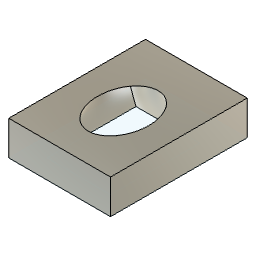
toothbrush_charger_case (Autodesk Fusion 360 design; units mm, degrees)
Autodesk Fusion 360 part; units mm, degrees
sketch "Sketch1" plane through (0, 0, 0) normal (0, 0, 1) x (1, 0, 0)
  line L0 (0, 0) -> (-70, 0)
  line L1 (-70, 0) -> (-70, 90)
  line L2 (-70, 90) -> (0, 90)
  line L3 (0, 90) -> (0, 0)
  line L4 (-70, 0) -> (0, 0)
  line L5 (0, 0) -> (0, 10)
  line L6 (0, 10) -> (-70, 10)
  line L7 (-70, 10) -> (-70, 0)
  line L8 (-70, 10) -> (-35, 10)
  line L9 (0, 10) -> (0, 32.5)
  line L10 (-35, 10) -> (-15, 10)
  line L11 (-15, 10) -> (-15, 37.5)
  line L12 (-15, 10) -> (-35, 10)
  line L13 (-35, 10) -> (-35, 37.5)
  line L14 (-35, 37.5) -> (-15, 37.5)
  line L15 (-15, 37.5) -> (-15, 10)
  ellipse E0 centre (-35, 37.5) end of major axis (-35, 10) minor radius 20
  line L16 (-35, 65) -> (-35, 10) construction
  line L17 (-55, 37.5) -> (-15, 37.5) construction
  line L18 (0, 10) -> (-10, 10)
  line L19 (-10, 10) -> (-60, 10)
  line L20 (-60, 10) -> (-60, 72.5)
  line L21 (-60, 72.5) -> (-10, 72.5)
  line L22 (-10, 72.5) -> (-10, 10)
  line L23 (0, 10) -> (-70, 10)
  line L24 (-70, 10) -> (-70, 2.5)
  line L25 (-70, 2.5) -> (0, 2.5)
  line L26 (0, 2.5) -> (0, 10)
  line L27 (0, 2.5) -> (-70, 2.5)
  line L28 (-70, 2.5) -> (-70, -7.5)
  line L29 (-70, -7.5) -> (0, -7.5)
  line L30 (0, -7.5) -> (0, 2.5)
  line L31 (-10, 10) -> (-60, 10)
  line L32 (-60, 10) -> (-60, 2.5)
  line L33 (-60, 2.5) -> (-10, 2.5)
  line L34 (-10, 2.5) -> (-10, 10)
  line L35 (0, -7.5) -> (5, -7.5)
  line L36 (5, -7.5) -> (5, -12.5)
  line L37 (5, -12.5) -> (0, -12.5)
  line L38 (0, -12.5) -> (0, -7.5)
  line L39 (5, -12.5) -> (-75, -12.5)
  line L40 (-75, -12.5) -> (-75, 95)
  line L41 (-75, 95) -> (5, 95)
  line L42 (5, 95) -> (5, -12.5)
  dimension "d1" = 70
  dimension "d2" = 90
  dimension "d3" = 10
  dimension "d4" = 35
  dimension "d5" = 22.5
  dimension "d6" = 20
  dimension "d7" = 27.5
  dimension "d8" = 27.5
  dimension "d11" = 10
  dimension "d12" = 50
  dimension "d13" = 62.5
  dimension "d14" = 70
  dimension "d15" = 7.5
  dimension "d16" = 70
  dimension "d17" = 10
  dimension "d20" = 50
  dimension "d21" = 7.5
  dimension "d22" = 5
  dimension "d23" = 5
  dimension "d24" = 80
  dimension "d25" = 107.5
  constraint horizontal L0
  constraint vertical L1
  constraint horizontal L2
  constraint vertical L3
  constraint coincident L0.start L3.end
  constraint horizontal L4
  constraint vertical L5
  constraint horizontal L6
  constraint vertical L7
  constraint perpendicular L7 L8
  constraint perpendicular L6 L9
  constraint parallel L6 L10
  constraint perpendicular L10 L11
  constraint horizontal L12
  constraint vertical L13
  constraint horizontal L14
  constraint vertical L15
  constraint coincident E0 L16.start
  constraint coincident E0 L8.end
  constraint coincident E0 L17.start
  constraint coincident E0 L11.end
  constraint coincident L13.end L14.start
  constraint coincident L8.end L10.start
  constraint perpendicular L6 L16
  constraint coincident L11.end L14.end
  constraint perpendicular L9 L18
  constraint horizontal L19
  constraint vertical L20
  constraint horizontal L21
  constraint vertical L22
  constraint horizontal L23
  constraint vertical L24
  constraint horizontal L25
  constraint vertical L26
  constraint horizontal L27
  constraint vertical L28
  constraint horizontal L29
  constraint vertical L30
  constraint horizontal L31
  constraint vertical L32
  constraint horizontal L33
  constraint vertical L34
  constraint horizontal L35
  constraint vertical L36
  constraint horizontal L37
  constraint vertical L38
  constraint horizontal L39
  constraint vertical L40
  constraint horizontal L41
  constraint vertical L42
  measures "d1" distance of L0.start L0.end
  measures "d2" distance of L0.start L2.end
  measures "d3" distance of L0.end L6.end
  measures "d4" distance of L6.end L8.end
  measures "d5" distance of L5.end L9.end
  measures "d6" distance of L8.end L10.end
  measures "d7" distance of L10.end L11.end
  measures "d8" distance of L10.end L11.end
  measures "d11" distance of L5.end L18.end
  measures "d12" distance of L18.end L19.end
  measures "d13" distance of L18.end L21.end
  measures "d14" distance of L5.end L6.end
  measures "d15" distance of L5.end L25.end
  measures "d16" distance of L25.end L24.end
  measures "d17" distance of L25.end L29.end
  measures "d20" distance of L18.end L19.end
  measures "d21" distance of L18.end L33.end
  measures "d22" distance of L29.end L35.end
  measures "d23" distance of L29.end L37.end
  measures "d24" distance of L36.end L39.end
  measures "d25" distance of L36.end L41.end
extrude "Extrude1" add sketch "Sketch1" along normal blind 27 contours L0 L1 L3 L4 L5 L7 L25 L27 L28 L30 L33 | L3 L5 L6 L18 L23 L25 L26 L27 L34 | L1 L6 L7 L8 L23 L24 L25 L27 L32 | L1 L2 L3 L6 L8 L9 L18 L20 L21 L22 L23 | L6 L8 L10 L12 L19 L23 L25 L27 L31 L32 L33 L34 | L6 L8 L11 L15 E0 L19 L20 L21 L22 L23 L31 | L6 L10 L11 L12 L15 E0 L19 L23 L31
extrude "Extrude2" add sketch "Sketch1" along normal blind 27 contours L0 L4 L28 L29 L30
sketch "Sketch2" plane through (0, 0, 27) normal (0, 0, 1) x (-1, 0, 0)
  ellipse E0 centre (35, -37.5) end of major axis (35, -10) minor radius 20
  line L0 (70, -90) -> (70, 7.5)
  line L1 (70, 7.5) -> (0, 7.5)
  line L2 (0, 7.5) -> (0, -90)
  line L3 (0, -90) -> (70, -90)
  ellipse E1 centre (35, -37.5) end of major axis (35, -10) minor radius 20
  line L4 (35, -65) -> (35, -10) construction
  line L5 (55, -37.5) -> (15, -37.5) construction
  constraint coincident E1 L4.start
  constraint coincident E1 L4.end
  constraint coincident E1 L5.start
  constraint coincident E1 L5.end
  constraint concentric E0 E1
  constraint vertical L4
loft "Loft1" cut profiles "Sketch2", "Sketch1" section 1 contours E0 E1 section 2 contours L6 L8 L10 L12 L19 L23 L25 L27 L31 L32 L33 L34 | L6 L8 L11 L15 E0 L19 L20 L21 L22 L23 L31 | L6 L10 L11 L12 L15 E0 L19 L23 L31
extrude "Extrude3" add sketch "Sketch1" along normal blind 27
sketch "Sketch3" plane through (0, 0, 0) normal (0, 0, -1) x (1, 0, 0)
  line L0 (-75, -95) -> (5, -95)
  line L1 (5, -95) -> (5, 12.5)
  line L2 (5, 12.5) -> (-75, 12.5)
  line L3 (-75, 12.5) -> (-75, -95)
  line L4 (-60, -72.5) -> (-60, -2.5)
  line L5 (-60, -2.5) -> (-10, -2.5)
  line L6 (-10, -2.5) -> (-10, -72.5)
  line L7 (-10, -72.5) -> (-60, -72.5)
  measures "d8" distance of origin
